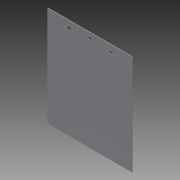
# Autodesk Inventor part: prototype build plate large
Saved by Autodesk Inventor 2014 SP1 (Build 180222100, 222)
## iProperties
Created: 2014-10-08
Part Number: prototype build plate large
Material: Aluminum 6061
Document SubType Name: Modeling
Designer: Mon
Density: 2.71 g/cm^3
Appearance: Aluminum - Flat
Author: Mon
Autodesk Inventor part; units mm, degrees
ref_plane "YZ Plane" through (0, 0, 0) normal (1, 0, 0) x (0, 1, 0)
ref_plane "XZ Plane" through (0, 0, 0) normal (0, 1, 0) x (-1, 0, 0)
ref_plane "XY Plane" through (0, 0, 0) normal (0, 0, 1) x (1, 0, 0)
sketch "Sketch9" plane through (0, 0, 0) normal (0, 1, 0) x (-1, 0, 0)
  line L0 (0, 0) -> (304.8, 0)
  line L1 (304.8, 0) -> (304.8, -360)
  line L2 (304.8, -360) -> (0, -360)
  line L3 (0, -360) -> (0, 0)
  line L4 (152.4, 0) -> (152.4, -19) construction
  circle A0 centre (152.4, -19) radius 5
  line L5 (20.9546, -25) -> (290.8502, -25) construction
  line L6 (152.4, 0) -> (227.4, 0) construction
  line L7 (227.4, -43.4011) -> (227.4, 0) construction
  line L8 (152.4, 0) -> (77.4, 0) construction
  line L9 (77.4, -41.0151) -> (77.4, 0) construction
  circle A1 centre (77.4, -25) radius 6
  circle A2 centre (227.4, -25) radius 6
  circle A3 centre (77.4, -25) radius 14 construction
  circle A4 centre (77.4, -11) radius 2
  circle A5 centre (91.4, -25) radius 2
  circle A6 centre (77.4, -39) radius 2
  circle A7 centre (63.4, -25) radius 2
  circle A8 centre (227.4, -25) radius 14 construction
  circle A9 centre (227.4, -11) radius 2
  circle A10 centre (241.4, -25) radius 2
  circle A11 centre (227.4, -39) radius 2
  circle A12 centre (213.4, -25) radius 2
  dimension "d22" = 304.8
  dimension "d23" = 360
  dimension "d24" = 19
  dimension "d25" = 10
  dimension "d27" = 12
  dimension "d28" = 12
  dimension "d30" = 28
  dimension "d31" = 4
  dimension "d32" = 4
  dimension "d33" = 4
  dimension "d34" = 4
  dimension "d35" = 75
  dimension "d36" = 11
  dimension "d37" = 77.4
  dimension "d38" = 25
  dimension "d39" = 28
  dimension "d40" = 4
  dimension "d41" = 4
  dimension "d42" = 4
  dimension "d43" = 4
  dimension "d44" = 11
  constraints: 20 end point, 13 centre point, 12 point on line, 8 point on circle, 3 coincident, 3 parallel, 3 perpendicular, 1 horizontal, 1 midpoint
  measures "d22" distance of L1.end L2.end
  measures "d23" distance of L0.end L1.end
  measures "d24" distance of L4.start L4.end
  measures "d25" diameter of A0
  measures "d27" diameter of A1
  measures "d28" diameter of A2
  measures "d30" diameter of A3
  measures "d31" diameter of A4
  measures "d32" diameter of A5
  measures "d33" diameter of A6
  measures "d34" diameter of A7
  measures "d35" distance of L8.end L4.start
  measures "d36" distance of A4.centre L8.end
  measures "d37" distance from line of L1 A2.centre
  measures "d38" distance between parallel lines of L5 L0
  measures "d39" diameter of A8
  measures "d40" diameter of A9
  measures "d41" diameter of A10
  measures "d42" diameter of A11
  measures "d43" diameter of A12
  measures "d44" distance of L6.end A9.centre
extrude "Extrusion5" add sketch "Sketch9" along normal blind 1.5875
body "Solid2"
